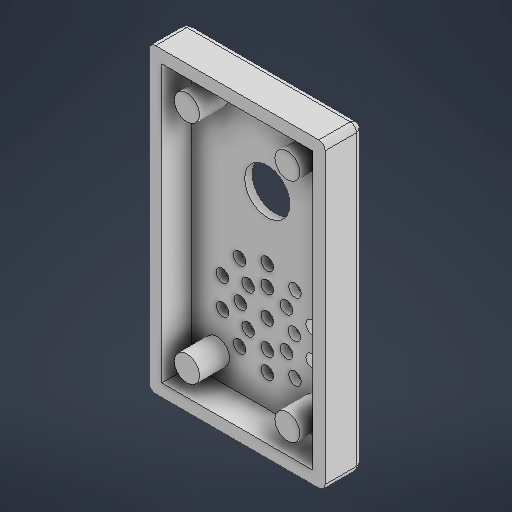
# Autodesk Inventor part: Top_Shell
Saved by Autodesk Inventor 2026.2 (Build 302298010, 298A)
## iProperties
Created: 2026-03-03
Part Number: Top_Shell
Material: Generic
Document SubType Name: Modeling
Designer: kjedr
Density: 1 g/cm^3
Appearance: Default
Author: kjedr
Autodesk Inventor part; units mm, degrees
ref_plane "YZ Plane" through (0, 0, 0) normal (1, 0, 0) x (0, 1, 0)
ref_plane "XZ Plane" through (0, 0, 0) normal (0, 1, 0) x (-1, 0, 0)
ref_plane "XY Plane" through (0, 0, 0) normal (0, 0, 1) x (1, 0, 0)
sketch "Sketch1" plane through (0, 0, 0) normal (0, 0, 1) x (1, 0, 0)
  line L0 (0, 0) -> (88.9, 0)
  line L1 (88.9, 0) -> (88.9, 152.4)
  line L2 (88.9, 152.4) -> (0, 152.4)
  line L3 (0, 152.4) -> (0, 0)
  dimension "d0" = 88.9
  dimension "d1" = 152.4
  constraints: 8 end point, 2 parallel, 1 horizontal, 1 perpendicular
  measures "d0" distance of L2.end L1.end
  measures "d1" distance of L1.end L0.end
extrude "Extrusion1" add sketch "Sketch1" along normal blind 19.05
sketch "Sketch2" plane through (0, 0, 19.05) normal (0, 0, 1) x (1, 0, 0)
  line L0 (6.35, 6.35) -> (82.55, 6.35)
  line L1 (82.55, 6.35) -> (82.55, 146.05)
  line L2 (82.55, 146.05) -> (6.35, 146.05)
  line L3 (6.35, 146.05) -> (6.35, 6.35)
  line L4 (0, 152.4) -> (0, 0) projected
  line L5 (0, 0) -> (88.9, 0) projected
  line L6 (88.9, 0) -> (88.9, 152.4) projected
  line L7 (88.9, 152.4) -> (0, 152.4) projected
  point P0 (88.9, 76.2)
  dimension "d4" = 6.35
  dimension "d5" = 6.35
  dimension "d6" = 6.35
  dimension "d7" = 6.35
  constraints: 8 end point, 2 parallel, 1 horizontal, 1 midpoint, 1 perpendicular
  measures "d4" distance between parallel lines of L4 L3
  measures "d5" distance between parallel lines of L5 L0
  measures "d6" distance from line of point (88.9, 76.2) L1
  measures "d7" distance between parallel lines of L7 L2
extrude "Extrusion2" cut sketch "Sketch2" against normal blind 15.24 contours L3 L2 L1 L0
sketch "Sketch3" plane through (0, 0, 3.81) normal (0, 0, 1) x (1, 0, 0)
  circle A0 centre (19.05, 133.35) radius 6.35
  circle A1 centre (69.85, 133.35) radius 6.35
  circle A2 centre (19.05, 19.05) radius 6.35
  circle A3 centre (69.85, 19.05) radius 6.35
  line L0 (6.35, 6.35) -> (6.35, 146.05) projected
  line L1 (6.35, 146.05) -> (82.55, 146.05) projected
  line L2 (82.55, 6.35) -> (6.35, 6.35) projected
  line L3 (82.55, 146.05) -> (82.55, 6.35) projected
  point P0 (0, 0)
  dimension "d10" = 12.7
  dimension "d11" = 12.7
  dimension "d12" = 12.7
  dimension "d13" = 12.7
  dimension "d14" = 12.7
  constraints: 4 centre point, 3 equal radius, 2 horizontal alignment, 2 vertical alignment
  measures "d10" distance from line of L0 A0.centre
  measures "d11" distance from line of L1 A0.centre
  measures "d12" distance from line of L2 A2.centre
  measures "d13" distance from line of L3 A1.centre
  measures "d14" diameter of A0
extrude "Extrusion3" add sketch "Sketch3" along normal up to surface (15.24 mm away) contours A0 | A1 | A2 | A3
fillet "Fillet1" radius 3.175 8 edges at (88.9, 152.4, 9.525) (0, 152.4, 9.525) (44.45, 152.4, 0) (88.9, 76.2, 0) (44.45, 0, 0) (0, 76.2, 0) (0, 0, 9.525) (88.9, 0, 9.525)
sketch "Sketch6" plane through (0, 0, 0) normal (0, 0, -1) x (-1, 0, 0)
  circle A0 centre (-44.45, 101.6) radius 11.43
  line L0 (-85.725, 149.225) -> (-3.175, 149.225) projected
  line L1 (-3.175, 152.4) -> (-85.725, 152.4) projected
  point P0 (0, 0)
  point P1 (-44.45, 149.225)
  dimension "d18" = 22.86
  dimension "d19" = 50.8
  constraints: 1 centre point, 1 midpoint, 1 vertical alignment
  measures "d18" diameter of A0
  measures "d19" distance from line of L1 A0.centre
extrude "Extrusion4" cut sketch "Sketch6" against normal through all
sketch "Sketch7" plane through (0, 0, 0) normal (0, 0, -1) x (-1, 0, 0)
  circle A0 centre (-44.45, 46.1045) radius 23.8125 construction
  circle A1 centre (-44.45, 69.917) radius 3.175
  circle A2 centre (-58.4466, 65.3692) radius 3.175
  circle A3 centre (-67.097, 53.4629) radius 3.175
  circle A4 centre (-67.097, 38.746) radius 3.175
  circle A5 centre (-58.4466, 26.8398) radius 3.175
  circle A6 centre (-44.45, 22.292) radius 3.175
  circle A7 centre (-30.4534, 26.8398) radius 3.175
  circle A8 centre (-21.803, 38.746) radius 3.175
  circle A9 centre (-21.803, 53.4629) radius 3.175
  circle A10 centre (-30.4534, 65.3692) radius 3.175
  circle A11 centre (-44.45, 46.1045) radius 13.6525 construction
  circle A12 centre (-44.45, 59.757) radius 3.175
  circle A13 centre (-44.45, 46.1045) radius 13.6525 construction
  circle A14 centre (-54.1038, 55.7582) radius 3.175
  circle A15 centre (-44.45, 46.1045) radius 13.6525 construction
  circle A16 centre (-58.1025, 46.1045) radius 3.175
  circle A17 centre (-44.45, 46.1045) radius 13.6525 construction
  circle A18 centre (-54.1038, 36.4507) radius 3.175
  circle A19 centre (-44.45, 46.1045) radius 13.6525 construction
  circle A20 centre (-44.45, 32.452) radius 3.175
  circle A21 centre (-44.45, 46.1045) radius 13.6525 construction
  circle A22 centre (-34.7962, 36.4507) radius 3.175
  circle A23 centre (-44.45, 46.1045) radius 13.6525 construction
  circle A24 centre (-30.7975, 46.1045) radius 3.175
  circle A25 centre (-44.45, 46.1045) radius 13.6525 construction
  circle A26 centre (-34.7962, 55.7582) radius 3.175
  circle A27 centre (-44.45, 46.1045) radius 3.175
  point P0 (0, 0)
  dimension "d22" = 47.625
  dimension "d28" = 10.16
  dimension "d23" = 6.35
  dimension "d26" = 360
  dimension "d29" = 6.35
  dimension "d32" = 360
  dimension "d34" = 6.35
  constraints: 19 centre point, 3 vertical alignment, 2 coincident, 2 horizontal alignment, 76 other
  measures "d23" diameter of A1
  measures "d29" diameter of A12
  measures "d34" diameter of A27
extrude "Extrusion5" cut sketch "Sketch7" against normal through all
body "Solid1"
